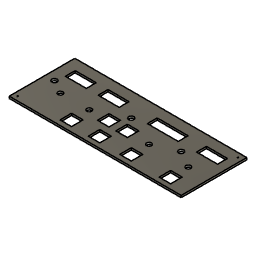
fcu-panel-SOURCEFILE v1 (Autodesk Fusion 360 design; units mm, degrees)
Autodesk Fusion 360 part; units mm, degrees
sketch "Sketch1" plane through (0, 0, 0) normal (0, 0, 1) x (1, 0, 0)
  line L0 (0, 0) -> (262, 0)
  line L1 (262, 0) -> (262, 100.0014)
  line L2 (262, 100.0014) -> (0, 100.0014)
  line L3 (0, 100.0014) -> (0, 0)
  constraint horizontal L0
  constraint vertical L1
  constraint horizontal L2
  constraint vertical L3
  constraint coincident L0.start L3.end
extrude "Extrude1" add sketch "Sketch1" along normal blind 3
sketch "Sketch2" plane through (0, 0, 3) normal (0, 0, 1) x (-1, 0, 0)
  line L0 (0, -100.0014) -> (0, 0)
  line L1 (0, 0) -> (-262, 0)
  line L2 (-262, 0) -> (-262, -100.0014)
  line L3 (-262, -100.0014) -> (0, -100.0014)
  line L4 (-141.5, -69) -> (-141.5, -84)
  line L5 (-188.5, -84) -> (-188.5, -69)
  line L6 (-141.5, -84) -> (-188.5, -84)
  line L7 (-188.5, -69) -> (-141.5, -69)
  line L8 (-216.5, -84) -> (-248.5, -84)
  line L9 (-216.5, -69) -> (-216.5, -84)
  line L10 (-248.5, -69) -> (-216.5, -69)
  line L11 (-248.5, -84) -> (-248.5, -69)
  line L12 (-16.5, -84) -> (-48.5, -84)
  line L13 (-48.5, -84) -> (-48.5, -69)
  line L14 (-16.5, -69) -> (-16.5, -84)
  line L15 (-48.5, -69) -> (-16.5, -69)
  line L16 (-98.5, -69) -> (-66.5, -69)
  line L17 (-98.5, -84) -> (-98.5, -69)
  line L18 (-66.5, -84) -> (-98.5, -84)
  line L19 (-66.5, -69) -> (-66.5, -84)
  line L20 (-113, -25) -> (-130.6, -25)
  line L21 (-130.6, -25) -> (-130.6, -7.4)
  line L22 (-130.6, -7.4) -> (-113, -7.4)
  line L23 (-113, -7.4) -> (-113, -25)
  line L24 (-144.6, -53) -> (-144.6, -35.4)
  line L25 (-127, -53) -> (-144.6, -53)
  line L26 (-127, -35.4) -> (-127, -53)
  line L27 (-144.6, -35.4) -> (-127, -35.4)
  line L28 (-116.6, -53) -> (-116.6, -35.4)
  line L29 (-99, -53) -> (-116.6, -53)
  line L30 (-99, -35.4) -> (-99, -53)
  line L31 (-116.6, -35.4) -> (-99, -35.4)
  circle A0 centre (-35, -43) radius 3.8
  circle A1 centre (-79, -43) radius 3.8
  circle A2 centre (-170, -43) radius 3.8
  circle A3 centre (-230, -43) radius 3.8
  circle A4 centre (-122, -64) radius 4
  circle A5 centre (-14, -55) radius 4
  circle A6 centre (-204, -58) radius 4
  line L32 (-87.6, -25) -> (-87.6, -7.4)
  line L33 (-70, -25) -> (-87.6, -25)
  line L34 (-70, -7.4) -> (-70, -25)
  line L35 (-87.6, -7.4) -> (-70, -7.4)
  line L36 (-178.6, -25) -> (-178.6, -7.4)
  line L37 (-161, -25) -> (-178.6, -25)
  line L38 (-161, -7.4) -> (-161, -25)
  line L39 (-178.6, -7.4) -> (-161, -7.4)
  line L40 (-238.6, -25) -> (-238.6, -7.4)
  line L41 (-221, -25) -> (-238.6, -25)
  line L42 (-221, -7.4) -> (-221, -25)
  line L43 (-238.6, -7.4) -> (-221, -7.4)
  point P0 (-56, -93.0014)
  dimension "d15" = 47
  dimension "d16" = 15
  dimension "d17" = 32
  dimension "d18" = 15
  dimension "d19" = 32
  dimension "d20" = 15
  dimension "d21" = 32
  dimension "d22" = 15
  dimension "d24" = 17.6
  dimension "d25" = 17.6
  dimension "d26" = 17.6
  dimension "d27" = 17.6
  dimension "d28" = 17.6
  dimension "d29" = 17.6
  dimension "d31" = 7.6
  dimension "d32" = 7.6
  dimension "d33" = 7.6
  dimension "d34" = 7.6
  dimension "d35" = 8
  dimension "d36" = 8
  dimension "d37" = 8
  dimension "d38" = 17.6
  dimension "d39" = 17.6
  dimension "d40" = 17.6
  dimension "d41" = 17.6
  dimension "d42" = 17.6
  dimension "d43" = 17.6
  constraint horizontal L6
  constraint vertical L5
  constraint horizontal L7
  constraint vertical L4
  constraint horizontal L8
  constraint vertical L11
  constraint horizontal L10
  constraint vertical L9
  constraint horizontal L12
  constraint vertical L13
  constraint horizontal L15
  constraint vertical L14
  constraint horizontal L18
  constraint vertical L17
  constraint horizontal L16
  constraint vertical L19
  constraint horizontal L20
  constraint vertical L21
  constraint horizontal L22
  constraint vertical L23
  constraint horizontal L25
  constraint vertical L24
  constraint horizontal L27
  constraint vertical L26
  constraint horizontal L29
  constraint vertical L28
  constraint horizontal L31
  constraint vertical L30
  constraint horizontal L33
  constraint vertical L32
  constraint horizontal L35
  constraint vertical L34
  constraint horizontal L37
  constraint vertical L36
  constraint horizontal L39
  constraint vertical L38
  constraint horizontal L41
  constraint vertical L40
  constraint horizontal L43
  constraint vertical L42
  measures "d15" distance of L5.start L4.end
  measures "d16" distance of L4.start L4.end
  measures "d17" distance of L8.start L8.end
  measures "d18" distance of L8.start L9.start
  measures "d19" distance of L12.end L12.start
  measures "d20" distance of L14.start L12.start
  measures "d21" distance of L17.start L18.start
  measures "d22" distance of L16.end L18.start
  measures "d24" distance of L20.start L20.end
  measures "d25" distance of L20.start L22.end
  measures "d26" distance of L25.start L24.start
  measures "d27" distance of L25.start L26.start
  measures "d28" distance of L29.start L28.start
  measures "d29" distance of L29.start L30.start
  measures "d31" diameter of A0
  measures "d32" diameter of A1
  measures "d33" diameter of A2
  measures "d34" diameter of A3
  measures "d35" diameter of A4
  measures "d36" diameter of A5
  measures "d37" diameter of A6
  measures "d38" distance of L33.start L32.start
  measures "d39" distance of L33.start L34.start
  measures "d40" distance of L37.start L36.start
  measures "d41" distance of L37.start L38.start
  measures "d42" distance of L41.start L40.start
  measures "d43" distance of L41.start L42.start
extrude "Extrude2" cut sketch "Sketch2" against normal blind 20 contours L4 L5 L6 L7 | L8 L9 L10 L11 | L12 L13 L14 L15 | L16 L17 L18 L19 | L20 L21 L22 L23 | L24 L25 L26 L27 | L28 L29 L30 L31 | A0 | A1 | A2 | A3 | A4 | A5 | A6 | L32 L33 L34 L35 | L36 L37 L38 L39 | L40 L41 L42 L43
sketch "Sketch3" plane through (0, 0, 0) normal (0, 0, -1) x (1, 0, 0)
  circle A0 centre (170, -43) radius 3.8
  line L0 (216.5, -84) -> (216.5, -69)
  line L1 (216.5, -69) -> (248.5, -69)
  line L2 (248.5, -69) -> (248.5, -84)
  line L3 (248.5, -84) -> (216.5, -84)
  line L4 (130.6, -7.4) -> (130.6, -25)
  line L5 (130.6, -25) -> (113, -25)
  line L6 (113, -25) -> (113, -7.4)
  line L7 (113, -7.4) -> (130.6, -7.4)
  line L8 (98.5, -69) -> (98.5, -84)
  line L9 (98.5, -84) -> (66.5, -84)
  line L10 (66.5, -84) -> (66.5, -69)
  line L11 (66.5, -69) -> (98.5, -69)
  line L12 (116.6, -53) -> (99, -53)
  line L13 (99, -53) -> (99, -35.4)
  line L14 (99, -35.4) -> (116.6, -35.4)
  line L15 (116.6, -35.4) -> (116.6, -53)
  line L16 (87.6, -25) -> (70, -25)
  line L17 (70, -25) -> (70, -7.4)
  line L18 (70, -7.4) -> (87.6, -7.4)
  line L19 (87.6, -7.4) -> (87.6, -25)
  line L20 (188.5, -84) -> (141.5, -84)
  line L21 (141.5, -84) -> (141.5, -69)
  line L22 (141.5, -69) -> (188.5, -69)
  line L23 (188.5, -69) -> (188.5, -84)
  circle A1 centre (204, -58) radius 4
  circle A2 centre (35, -43) radius 3.8
  line L24 (238.6, -25) -> (221, -25)
  line L25 (221, -25) -> (221, -7.4)
  line L26 (221, -7.4) -> (238.6, -7.4)
  line L27 (238.6, -7.4) -> (238.6, -25)
  line L28 (144.6, -53) -> (127, -53)
  line L29 (127, -53) -> (127, -35.4)
  line L30 (127, -35.4) -> (144.6, -35.4)
  line L31 (144.6, -35.4) -> (144.6, -53)
  circle A3 centre (79, -43) radius 3.8
  circle A4 centre (122, -64) radius 4
  line L32 (48.5, -84) -> (16.5, -84)
  line L33 (16.5, -84) -> (16.5, -69)
  line L34 (16.5, -69) -> (48.5, -69)
  line L35 (48.5, -69) -> (48.5, -84)
  line L36 (178.6, -25) -> (161, -25)
  line L37 (161, -25) -> (161, -7.4)
  line L38 (161, -7.4) -> (178.6, -7.4)
  line L39 (178.6, -7.4) -> (178.6, -25)
  circle A5 centre (230, -43) radius 3.8
  circle A6 centre (14, -55) radius 4
  line L40 (0, 0) -> (0, -100.0014)
  line L41 (0, -100.0014) -> (262, -100.0014)
  line L42 (262, -100.0014) -> (262, 0)
  line L43 (262, 0) -> (0, 0)
  circle A7 centre (6.5, -6.5) radius 0.85
  dimension "d46" = 1.7
  measures "d46" diameter of A7
extrude "Extrude3" cut sketch "Sketch3" against normal blind 4 contours A7
sketch "Sketch4" plane through (0, 0, 0) normal (0, 0, -1) x (1, 0, 0)
  circle A0 centre (6.5, -6.5) radius 0.85
  circle A1 centre (170, -43) radius 3.8
  line L0 (216.5, -84) -> (216.5, -69)
  line L1 (216.5, -69) -> (248.5, -69)
  line L2 (248.5, -69) -> (248.5, -84)
  line L3 (248.5, -84) -> (216.5, -84)
  line L4 (130.6, -7.4) -> (130.6, -25)
  line L5 (130.6, -25) -> (113, -25)
  line L6 (113, -25) -> (113, -7.4)
  line L7 (113, -7.4) -> (130.6, -7.4)
  line L8 (98.5, -69) -> (98.5, -84)
  line L9 (98.5, -84) -> (66.5, -84)
  line L10 (66.5, -84) -> (66.5, -69)
  line L11 (66.5, -69) -> (98.5, -69)
  line L12 (116.6, -53) -> (99, -53)
  line L13 (99, -53) -> (99, -35.4)
  line L14 (99, -35.4) -> (116.6, -35.4)
  line L15 (116.6, -35.4) -> (116.6, -53)
  line L16 (87.6, -25) -> (70, -25)
  line L17 (70, -25) -> (70, -7.4)
  line L18 (70, -7.4) -> (87.6, -7.4)
  line L19 (87.6, -7.4) -> (87.6, -25)
  line L20 (188.5, -84) -> (141.5, -84)
  line L21 (141.5, -84) -> (141.5, -69)
  line L22 (141.5, -69) -> (188.5, -69)
  line L23 (188.5, -69) -> (188.5, -84)
  circle A2 centre (204, -58) radius 4
  circle A3 centre (35, -43) radius 3.8
  line L24 (238.6, -25) -> (221, -25)
  line L25 (221, -25) -> (221, -7.4)
  line L26 (221, -7.4) -> (238.6, -7.4)
  line L27 (238.6, -7.4) -> (238.6, -25)
  line L28 (144.6, -53) -> (127, -53)
  line L29 (127, -53) -> (127, -35.4)
  line L30 (127, -35.4) -> (144.6, -35.4)
  line L31 (144.6, -35.4) -> (144.6, -53)
  circle A4 centre (79, -43) radius 3.8
  circle A5 centre (122, -64) radius 4
  line L32 (48.5, -84) -> (16.5, -84)
  line L33 (16.5, -84) -> (16.5, -69)
  line L34 (16.5, -69) -> (48.5, -69)
  line L35 (48.5, -69) -> (48.5, -84)
  line L36 (178.6, -25) -> (161, -25)
  line L37 (161, -25) -> (161, -7.4)
  line L38 (161, -7.4) -> (178.6, -7.4)
  line L39 (178.6, -7.4) -> (178.6, -25)
  circle A6 centre (230, -43) radius 3.8
  circle A7 centre (14, -55) radius 4
  line L40 (0, 0) -> (0, -100.0014)
  line L41 (0, -100.0014) -> (262, -100.0014)
  line L42 (262, -100.0014) -> (262, 0)
  line L43 (262, 0) -> (0, 0)
  circle A8 centre (255.2, -93.2014) radius 0.85
  dimension "d49" = 1.7
  measures "d49" diameter of A8
extrude "Extrude4" cut sketch "Sketch4" against normal blind 5 contours A8
